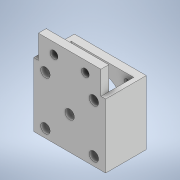
# Autodesk Inventor part: Base Motor Z
Saved by Autodesk Inventor 2021 (Build 250183000, 183)
## iProperties
Created: 2023-01-28
Part Number: Base Motor Z
Material: Genérico
Document SubType Name: Modeling
Designer: Diego.labarca
Density: 1 g/cm^3
Appearance: Valor por defecto
Author: Diego.labarca
Autodesk Inventor part; units mm, degrees
ref_plane "YZ Plane" through (0, 0, 0) normal (1, 0, 0) x (0, 1, 0)
ref_plane "XZ Plane" through (0, 0, 0) normal (0, 1, 0) x (-1, 0, 0)
sketch "Boceto1" plane through (0, 0, 0) normal (0, 0, 1) x (1, 0, 0)
  line L0 (-20, 20) -> (20, 20)
  line L1 (20, 20) -> (20, -20)
  line L2 (20, -20) -> (-20, -20)
  line L3 (-20, -20) -> (-20, 20)
  line L4 (6.44, 0) -> (0, 0)
  line L5 (0, 0) -> (0, 3.5859)
  dimension "d0" = 40
  dimension "d1" = 40
  constraints: 12 end point, 2 horizontal, 2 parallel, 2 perpendicular, 2 other
  measures "d0" distance of L1.end L2.end
  measures "d1" distance of L0.end L1.end
extrude "Extrusión1" add sketch "Boceto1" along normal blind 5
sketch "Boceto2" plane through (0, 0, 5) normal (0, 0, 1) x (1, 0, 0)
  circle A0 centre (15.5, 15.5) radius 1.5
  point P0 (0, 0)
  dimension "d4" = 3
  dimension "d5" = 15.5
  dimension "d6" = 15.5
  constraints: 1 centre point
  measures "d4" diameter of A0
  measures "d5" horizontal distance of point (0, 0) A0.centre
  measures "d6" horizontal distance of point (0, 0) A0.centre
extrude "Extrusión2" cut sketch "Boceto2" against normal through all
pattern_linear "Patrón rectangular1" count 2 spacing 31 along (-1, 0, 0) count 2 spacing 31 along (0, -1, 0) of "Extrusión2"
ref_plane "Plano de trabajo1" through (0, 0, 26) normal (0, 0, -1) x (-1, 0, 0)
sketch "Boceto6" plane through (0, 0, 26) normal (0, 0, -1) x (-1, 0, 0)
  circle A0 centre (15.5, -15.5) radius 1.5 projected
  circle A1 centre (-15.5, -15.5) radius 1.5 projected
  circle A2 centre (15.5, 15.5) radius 1.5 projected
  circle A3 centre (-15.5, 15.5) radius 1.5 projected
  line L0 (20, -20) -> (-20, -20) projected
  line L1 (-20, -20) -> (-20, 20) projected
  line L2 (-20, 20) -> (20, 20) projected
  line L3 (20, 20) -> (20, -20) projected
  line L4 (20, 20) -> (-20, 20)
  line L5 (-20, 20) -> (-20, 35)
  line L6 (-20, 35) -> (20, 35)
  line L7 (20, 35) -> (20, 20)
  circle A4 centre (-10, 28) radius 2.5
  circle A5 centre (10, 28) radius 2.5
  circle A6 centre (-15.5, -15.5) radius 3
  circle A7 centre (-15.5, 15.5) radius 1.5 projected
  circle A8 centre (-15.5, 15.5) radius 3
  circle A9 centre (15.5, 15.5) radius 1.5 projected
  circle A10 centre (15.5, 15.5) radius 3
  circle A11 centre (15.5, -15.5) radius 1.5 projected
  circle A12 centre (15.5, -15.5) radius 3
  dimension "d31" = 15
  dimension "d32" = 5
  dimension "d33" = 5
  dimension "d34" = 10
  dimension "d35" = 10
  dimension "d36" = 7
  dimension "d37" = 7
  dimension "d40" = 6
  dimension "d41" = 6
  dimension "d42" = 6
  dimension "d43" = 6
  constraints: 8 end point, 6 centre point, 4 coincident, 2 parallel, 1 horizontal, 1 perpendicular
  measures "d31" distance of L4.end L5.end
  measures "d32" diameter of A4
  measures "d33" diameter of A5
  measures "d34" distance from line of L5 A4.centre
  measures "d35" distance from line of L7 A5.centre
  measures "d36" distance from line of L6 A5.centre
  measures "d37" distance from line of L6 A4.centre
  measures "d40" diameter of A6
  measures "d41" diameter of A8
  measures "d42" diameter of A10
  measures "d43" diameter of A12
extrude "Extrusión5" add sketch "Boceto6" along normal blind 5 contours L0 L1 L2 L3 | L2 L5 L6 L7
sketch "Boceto7" plane through (-20, -20, 0) normal (-1, 0, 0) x (0, 0, 1)
  line L0 (26, 0) -> (26, 55) projected
  line L1 (5, 40) -> (5, 0) projected
  line L2 (5, 4) -> (21, 4)
  line L3 (21, 4) -> (21, -1)
  line L4 (21, -1) -> (5, -1)
  line L5 (5, -1) -> (5, 4)
  line L6 (26, 0) -> (21, 0) projected
  line L7 (0, 0) -> (5, 0) projected
  line L8 (5, -1) -> (0, -1)
  line L9 (0, -1) -> (0, 0)
  line L10 (0, 0) -> (5, 0)
  line L11 (5, 0) -> (5, -1)
  line L12 (21, -1) -> (26, -1)
  line L13 (26, -1) -> (26, 0)
  line L14 (26, 0) -> (21, 0)
  line L15 (21, 0) -> (21, -1)
  point P0 (0, 20)
  dimension "d48" = 1
  dimension "d49" = 5
  constraints: 24 end point, 6 parallel, 3 horizontal, 3 perpendicular, 1 point on line
  measures "d48" distance between parallel lines of L4 L6
  measures "d49" distance between parallel lines of L2 L4
extrude "Extrusión6" add sketch "Boceto7" against normal up to surface (40 mm away)
sketch "Boceto8" plane through (0, 0, 26) normal (0, 0, 1) x (1, 0, 0)
  circle A0 centre (-15.5, -15.5) radius 3 projected
  circle A1 centre (15.5, -15.5) radius 3 projected
  point P0 (0, 0)
extrude "Extrusión7" cut sketch "Boceto8" against normal up to surface (21 mm away)
sketch "Boceto9" plane through (-12.542, -16, 5) normal (0, 1, 0) x (1, 0, 0)
  circle A0 centre (2.542, -10) radius 2.5
  circle A1 centre (22.542, -10) radius 2.5
  line L0 (-7.458, -16) -> (-7.458, 0) projected
  line L1 (32.542, -16) -> (32.542, 0) projected
  line L2 (-7.458, -21) -> (32.542, -21) projected
  point P0 (12.542, 5)
  dimension "d52" = 5
  dimension "d53" = 5
  dimension "d54" = 10
  dimension "d55" = 10
  dimension "d56" = 11
  dimension "d57" = 11
  constraints: 2 centre point
  measures "d52" diameter of A0
  measures "d53" diameter of A1
  measures "d54" distance from line of L0 A0.centre
  measures "d55" distance from line of L1 A1.centre
  measures "d56" distance from line of L2 A0.centre
  measures "d57" distance from line of L2 A1.centre
extrude "Extrusión8" cut sketch "Boceto9" against normal through all
sketch "Boceto10" plane through (0, 0, 0) normal (0, 0, -1) x (-1, 0, 0)
  circle A0 centre (0, 0) radius 12.5
  dimension "d60" = 25
  constraints: 1 centre point, 1 coincident
  measures "d60" diameter of A0
extrude "Extrusión9" cut sketch "Boceto10" against normal up to surface (5 mm away)
sketch "Boceto11" plane through (-20, 20, 0) normal (0, 1, 0) x (1, 0, 0)
  line L0 (40, 0) -> (0, 0) projected
  line L1 (0, 0) -> (-3, 0)
  line L2 (-3, 0) -> (-3, -26)
  line L3 (-3, -26) -> (0, -26)
  line L4 (0, -26) -> (0, 0)
  line L5 (40, -26) -> (40, -21) projected
  line L6 (40, -26) -> (43, -26)
  line L7 (43, -26) -> (43, 0)
  line L8 (43, 0) -> (40, 0)
  line L9 (40, 0) -> (40, -26)
  point P0 (20, 0)
  dimension "d63" = 3
  dimension "d64" = 3
  constraints: 16 end point, 4 parallel, 2 horizontal, 2 perpendicular
  measures "d63" distance of L3.end L2.end
  measures "d64" distance of L8.end L7.end
extrude "Extrusión10" add sketch "Boceto11" against normal up to surface (41 mm away)
sketch "Boceto12" plane through (0, 0, 0) normal (0, 0, -1) x (-1, 0, 0)
  circle A0 centre (0, 0) radius 3
  dimension "d67" = 6
  constraints: 1 centre point, 1 coincident
  measures "d67" diameter of A0
extrude "Extrusión11" cut sketch "Boceto12" against normal up to surface (26 mm away)
equation "\"d33\" = d32"
equation "\"d35\" = d34"
equation "\"d36\" = d37"
equation "\"d41\" = d40"
equation "\"d42\" = d40"
equation "\"d43\" = d40"
equation "\"d53\" = d52"
equation "\"d57\" = d56"
equation "\"d64\" = d63"
